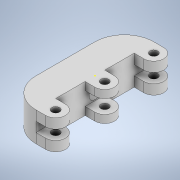
# Autodesk Inventor part: stuur_arm v2
Saved by Autodesk Inventor 2022 (Build 260153000, 153)
## iProperties
Created: 2021-12-08
Part Number: stuur_arm v2
Material: Generic
Document SubType Name: Modeling
Designer: keemi
Density: 1 g/cm^3
Appearance: Default
Author: keemi
## iProperties of the stored document stuur_arm v2_3DPrint.ipt
Created: 2021-12-09
Part Number: stuur_arm v2_3DPrint
Material: Generic
Document SubType Name: Modeling
Designer: keemi
Density: 1 g/cm^3
Appearance: Default
Author: keemi
Autodesk Inventor part; units mm, degrees
ref_plane "YZ Plane" through (0, 0, 0) normal (1, 0, 0) x (0, 1, 0)
ref_plane "XZ Plane" through (0, 0, 0) normal (0, 1, 0) x (-1, 0, 0)
ref_plane "XY Plane" through (0, 0, 0) normal (0, 0, 1) x (1, 0, 0)
sketch "Sketch1" plane through (0, 0, 0) normal (0, 1, 0) x (-1, 0, 0)
  line L0 (0, 0) -> (15, 0)
  line L1 (0, 0) -> (15, 0) construction
  line L2 (15, 0) -> (0, 0)
  line L3 (0, 0) -> (0, -30)
  line L4 (0, -30) -> (15, -30)
  line L5 (15, -30) -> (15, 0)
  line L6 (15, 0) -> (0, 0)
  line L7 (0, 0) -> (0, 30)
  line L8 (0, 30) -> (15, 30)
  line L9 (15, 30) -> (15, 0)
  dimension "d0" = 15
  dimension "d1" = 0
  dimension "d2" = 15
  dimension "d3" = 30
  dimension "d4" = 15
  dimension "d5" = 30
  constraints: 20 end point, 4 horizontal, 4 parallel, 2 perpendicular, 1 collinear
  measures "d0" distance of L0.start L0.end
  measures "d1" distance between parallel lines of L0 L1
  measures "d2" distance of L4.end L3.end
  measures "d3" distance of L3.end L2.end
  measures "d4" distance of L7.end L8.end
  measures "d5" distance of L6.end L7.end
extrude "Extrusion1" add sketch "Sketch1" against normal blind 15
fillet "Fillet1" radius 15 1 edges at (-15, -7.5, 30)
fillet "Fillet2" radius 15 1 edges at (-15, -7.5, -30)
sketch "Sketch2" plane through (-15, -15, 15) normal (-1, 0, 0) x (0, 0, 1)
  line L0 (-15, 15) -> (-15, 7.5)
  circle A0 centre (-15, 7.5) radius 3
  dimension "d10" = 7.5
  dimension "d11" = 6
  constraints: 2 end point, 1 centre point, 1 coincident, 1 vertical
  measures "d10" distance of L0.start L0.end
  measures "d11" diameter of A0
extrude "Extrusion2" cut sketch "Sketch2" against normal blind 15
sketch "Sketch3" plane through (0, -15, 30) normal (1, 0, 0) x (0, 0, -1)
  line L0 (30, 15) -> (30, 11)
  line L1 (60, 0) -> (0, 0) projected
  line L2 (40.1766, 0) -> (36.1766, 0)
  line L3 (40.1766, 0) -> (44.1766, 0) construction
  line L4 (30, 11) -> (35, 11)
  line L5 (60, 15) -> (60, 0) projected
  line L6 (0, 15) -> (60, 15) projected
  line L7 (50, 11) -> (60, 11)
  line L8 (60, 11) -> (60, 15)
  line L9 (60, 15) -> (50, 15)
  line L10 (50, 15) -> (50, 11)
  line L11 (50, 4) -> (60, 4)
  line L12 (60, 4) -> (60, 0)
  line L13 (60, 0) -> (50, 0)
  line L14 (0, 15) -> (0, 0) projected
  line L15 (40.1766, 4) -> (80.3532, 4) construction
  line L16 (30, 11) -> (0, 11)
  line L17 (0, 0) -> (10, 0)
  line L18 (10, 0) -> (10, 5)
  line L19 (10, 5) -> (0, 5)
  line L20 (0, 5) -> (0, 0)
  line L21 (0, 15) -> (10, 15)
  line L22 (10, 15) -> (10, 10)
  line L23 (10, 10) -> (0, 10)
  line L24 (0, 10) -> (0, 15)
  line L25 (35, 11) -> (25, 11)
  line L26 (25, 11) -> (25, 15)
  line L27 (25, 15) -> (35, 15)
  line L28 (35, 15) -> (35, 11)
  line L29 (60, 0) -> (50, 0)
  line L30 (50, 0) -> (50, 5)
  line L31 (50, 5) -> (60, 5)
  line L32 (60, 5) -> (60, 0)
  line L33 (60, 15) -> (50, 15)
  line L34 (50, 15) -> (50, 10)
  line L35 (50, 10) -> (60, 10)
  line L36 (60, 10) -> (60, 15)
  line L37 (30, 15) -> (30, -0.3417)
  line L38 (30, 0) -> (35, 0)
  line L39 (35, 0) -> (25, 0)
  line L40 (25, 0) -> (25, 4)
  line L41 (25, 4) -> (35, 4)
  line L42 (35, 4) -> (35, 0)
  point P0 (60, 5)
  point P1 (50, 0)
  point P2 (25, 15)
  point P3 (25, 11)
  dimension "d14" = 4
  dimension "d15" = 4
  dimension "d16" = 4
  dimension "d19" = 5
  dimension "d23" = 10
  dimension "d24" = 5
  dimension "d25" = 10
  dimension "d26" = 5
  dimension "d27" = 10
  dimension "d28" = 4
  dimension "d31" = 10
  dimension "d32" = 5
  dimension "d33" = 10
  dimension "d34" = 5
  dimension "d42" = 5
  dimension "d43" = 10
  dimension "d44" = 4
  constraints: 78 end point, 15 parallel, 11 horizontal, 9 perpendicular, 5 point on line, 2 vertical, 1 midpoint
  measures "d14" distance of L0.start L0.end
  measures "d15" distance of L2.start L2.end
  measures "d16" distance of L2.start L15.start
  measures "d19" distance of L0.end L4.end
  measures "d23" distance of L19.end L18.end
  measures "d24" distance of L18.end L17.end
  measures "d25" distance of L22.end L23.end
  measures "d26" distance of L21.end L22.end
  measures "d27" distance of L26.end L27.end
  measures "d28" distance of L25.end L26.end
  measures "d31" distance of L30.end L31.end
  measures "d32" distance of L29.end L30.end
  measures "d33" distance of L35.end L34.end
  measures "d34" distance of L34.end L33.end
  measures "d42" distance of L38.start L38.end
  measures "d43" distance of L40.end L41.end
  measures "d44" distance of L39.end L40.end
extrude "Extrusion3" add sketch "Sketch3" along normal blind 10 contours L6 L28 L4 L0 | L0 L16 L26 L6 | L41 L42 L1 L37 | L37 L1 L40 L41 | L22 L16 L14 L6 | L6 L5 L7 L10 | L22 L23 L14 L16 | L7 L5 L35 L34 | L1 L14 L19 L18 | L5 L11 L30 L31 | L30 L11 L5 L1
fillet "Fillet3" radius 5 12 edges at (10, -12.5, -30) (10, -2.5, -30) (10, -2.5, -20) (10, -12.5, -20) (10, -2, 5) (10, -2, -5) (10, -2.5, 20) (10, -2.5, 30) (10, -12.5, 20) (10, -12.5, 30) (10, -13, -5) (10, -13, 5)
sketch "Sketch4" plane through (0, 0, 0) normal (0, 1, 0) x (1, 0, 0)
  arc A0 (5, 5.1766) -> (5, 15.1766) centre (5, 10.1766) ccw projected
  arc A1 (5, 20) -> (5, 30) centre (5, 25) ccw projected
  circle A2 centre (5, 25) radius 2
  arc A3 (5, -30) -> (5, -20) centre (5, -25) ccw projected
  circle A4 centre (5, -25) radius 2
  arc A5 (5, -5) -> (5, 5) centre (5, 0) ccw projected
  circle A6 centre (5, 0) radius 2
  point P0 (0, 0)
  point P1 (10, 25)
  dimension "d39" = 4
  dimension "d45" = 4
  constraints: 3 centre point, 3 coincident
  measures "d39" diameter of A2
  measures "d45" diameter of A6
extrude "Extrusion4" cut sketch "Sketch4" against normal blind 15
sketch "Sketch5" plane through (0, 0, 20) normal (1, 0, 0) x (0, 0, -1)
  point P0 (20, 0)
sketch "Sketch6" plane through (0, 0, 0) normal (0, 1, 0) x (1, 0, 0)
  point P0 (0, 0)
body "Solid1"
